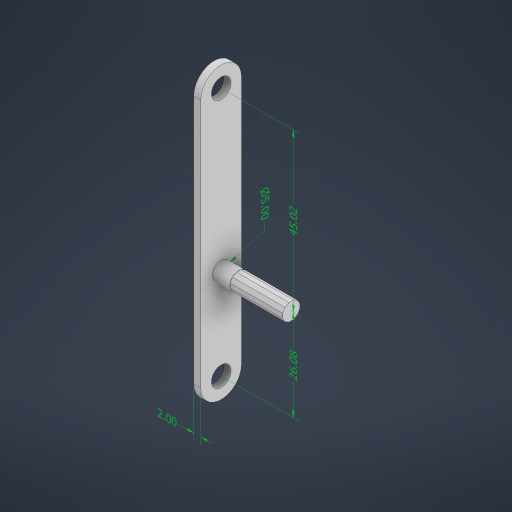
# Autodesk Inventor part: gunholder v2
Saved by Autodesk Inventor 2024 (Build 280153000, 153)
## iProperties
Created: 2023-06-17
Part Number: gunholder v2
Material: 일반
Document SubType Name: Modeling
Designer: 6gioc
Density: 1 g/cm^3
Appearance: 기본값
Mass: 1.95429 g
Surface Area: 23.4621 cm^2
Volume: 1.95429 cm^3
Author: 6gioc
## iProperties of the stored document gunholder v2_3D 인쇄.ipt
Created: 2023-06-20
Part Number: gunholder v2_3D 인쇄
Material: 일반
Document SubType Name: Modeling
Designer: 6gioc
Density: 1 g/cm^3
Appearance: 기본값
Author: 6gioc
Autodesk Inventor part; units mm, degrees
ref_plane "YZ Plane" through (0, 0, 0) normal (1, 0, 0) x (0, 1, 0)
ref_plane "XZ Plane" through (0, 0, 0) normal (0, 1, 0) x (-1, 0, 0)
ref_plane "XY Plane" through (0, 0, 0) normal (0, 0, 1) x (1, 0, 0)
sketch "스케치1" plane through (0, 0, 0) normal (1, 0, 0) x (0, 1, 0)
  circle A0 centre (71.1, 0) radius 2.8
  circle A1 centre (0, 0) radius 2.8
  circle A2 centre (71.1, 0) radius 5.8
  circle A3 centre (0, 0) radius 5.8
  line L0 (0, 5.8) -> (0, -5.8)
  line L1 (71.1, -5.8) -> (71.1, 5.8)
  line L2 (71.1, 5.8) -> (0, 5.8)
  line L3 (0, 5.8) -> (0, -5.8)
  line L4 (0, -5.8) -> (71.1, -5.8)
  line L5 (71.1, -5.8) -> (71.1, 5.8)
  circle A4 centre (26.083, 0) radius 2.5
  line L6 (28.4979, 0.647) -> (28.4979, -0.647)
  line L7 (28.4979, -0.647) -> (27.8508, -1.7678)
  line L8 (27.8508, -1.7678) -> (26.7301, -2.4148)
  line L9 (26.7301, -2.4148) -> (25.436, -2.4148)
  line L10 (25.436, -2.4148) -> (24.3153, -1.7678)
  line L11 (24.3153, -1.7678) -> (23.6682, -0.647)
  line L12 (23.6682, -0.647) -> (23.6682, 0.647)
  line L13 (23.6682, 0.647) -> (24.3153, 1.7678)
  line L14 (24.3153, 1.7678) -> (25.436, 2.4148)
  line L15 (25.436, 2.4148) -> (26.7301, 2.4148)
  line L16 (26.7301, 2.4148) -> (27.8508, 1.7678)
  line L17 (27.8508, 1.7678) -> (28.4979, 0.647)
  point P0 (28.583, 0)
  point P1 (23.6682, 0.647)
  point P2 (23.6682, 0.647)
  point P3 (28.4979, -0.647)
  point P4 (28.4979, -0.647)
  dimension "d6" = 11.6
  dimension "d14" = 5
  dimension "d2" = 5.6
  dimension "d3" = 5.6
  dimension "d5" = 11.6
  dimension "d8" = 11.6
  dimension "d9" = 71.1
  constraints: 36 end point, 5 coincident, 3 centre point, 3 parallel, 2 point on circle, 1 horizontal, 1 perpendicular, 32 other
  measures "d2" diameter of A0
  measures "d3" diameter of A1
  measures "d5" diameter of A2
  measures "d8" distance of L0.start L0.end
  measures "d9" distance of L0.end L4.end
extrude "돌출1" add sketch "스케치1" along normal blind 2 contours A0 L1 A2 | A0 L1 A2 | A2 L4 A3 L2 | L0 A1 A3 | A3 L0 A1
extrude "돌출2" add sketch "스케치1" along normal blind 7 contours A4 L6 | L17 A4 | L6 L7 L8 L9 L10 L11 L12 L13 L14 L15 L16 L17 | A4 L7 | L16 A4 | A4 L8 | L15 A4 | A4 L9 | L14 A4 | A4 L10 | L13 A4 | A4 L11 | L12 A4
extrude "돌출3" add sketch "스케치1" along normal blind 22 contours L6 L7 L8 L9 L10 L11 L12 L13 L14 L15 L16 L17
